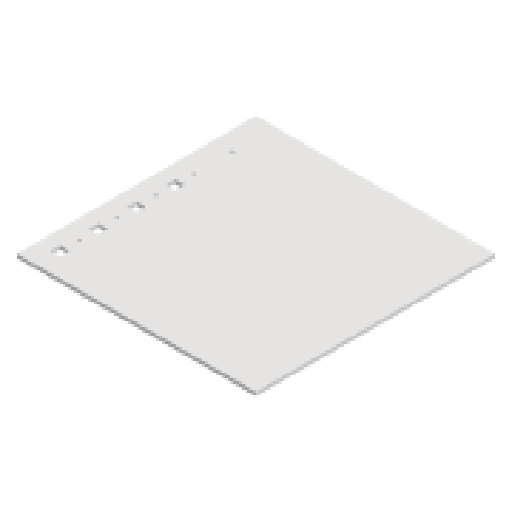
# Autodesk Inventor part: Платформа подъёмника
Saved by Autodesk Inventor 2023.2 (Build 272271030, 271C)
## iProperties
Created: 2025-03-18
Part Number: Платформа подъёмника
Material: Типовые
Document SubType Name: Modeling
Designer: Коноваленко
Density: 1 g/cm^3
Appearance: По умолчанию
Author: Коноваленко
Autodesk Inventor part; units mm, degrees
ref_plane "YZ Plane" through (0, 0, 0) normal (1, 0, 0) x (0, 1, 0)
ref_plane "XZ Plane" through (0, 0, 0) normal (0, 1, 0) x (-1, 0, 0)
ref_plane "XY Plane" through (0, 0, 0) normal (0, 0, 1) x (1, 0, 0)
sketch "Эскиз1" plane through (0, 0, 0) normal (0, 1, 0) x (-1, 0, 0)
  line L0 (125, 125) -> (-125, 125)
  line L1 (-125, 125) -> (-125, -125)
  line L2 (-125, -125) -> (125, -125)
  line L3 (125, -125) -> (125, 125)
  line L4 (125, 125) -> (-125, -125) construction
  line L5 (-125, 125) -> (125, -125) construction
  point P0 (0, 0)
  dimension "d0" = 250
  dimension "d1" = 250
  constraints: 12 end point, 2 midpoint, 2 parallel, 1 horizontal, 1 perpendicular
  measures "d0" distance of L1.end L2.end
  measures "d1" distance of L0.end L1.end
extrude "Выдавливание1" add sketch "Эскиз1" along normal blind 4
sketch "Эскиз2" plane through (0, 0, 0) normal (0, -1, 0) x (1, 0, 0)
  line L0 (-110, 90) -> (-110, 100) projected
  line L1 (-100, 90) -> (-110, 90) projected
  line L2 (-100, 100) -> (-100, 90) projected
  line L3 (-110, 100) -> (-100, 100) projected
  circle A0 centre (-105, 75) radius 2 projected
  circle A1 centre (-105, 35) radius 2 projected
  circle A2 centre (-105, -5) radius 2 projected
  circle A3 centre (-105, -45) radius 2 projected
  circle A4 centre (-105, -85) radius 2 projected
  line L4 (-110, 50) -> (-110, 60) projected
  line L5 (-100, 50) -> (-110, 50) projected
  line L6 (-100, 60) -> (-100, 50) projected
  line L7 (-110, 60) -> (-100, 60) projected
  line L8 (-110, 10) -> (-110, 20) projected
  line L9 (-100, 10) -> (-110, 10) projected
  line L10 (-100, 20) -> (-100, 10) projected
  line L11 (-110, 20) -> (-100, 20) projected
  line L12 (-110, -30) -> (-110, -20) projected
  line L13 (-100, -30) -> (-110, -30) projected
  line L14 (-100, -20) -> (-100, -30) projected
  line L15 (-110, -20) -> (-100, -20) projected
  line L16 (125, 125) -> (125, -125) projected
  line L17 (-125, 125) -> (125, 125) projected
  line L18 (-125, -125) -> (-125, 125) projected
  line L19 (125, -125) -> (-125, -125) projected
  line L20 (110, 90) -> (110, 100) projected
  line L21 (110, 100) -> (100, 100) projected
  line L22 (100, 100) -> (100, 90) projected
  line L23 (100, 90) -> (110, 90) projected
  line L24 (110, 10) -> (110, 20) projected
  line L25 (110, 20) -> (100, 20) projected
  line L26 (100, 20) -> (100, 10) projected
  line L27 (100, 10) -> (110, 10) projected
  line L28 (110, 50) -> (110, 60) projected
  line L29 (110, 60) -> (100, 60) projected
  line L30 (100, 60) -> (100, 50) projected
  line L31 (100, 50) -> (110, 50) projected
  line L32 (110, -30) -> (110, -20) projected
  line L33 (110, -20) -> (100, -20) projected
  line L34 (100, -20) -> (100, -30) projected
  line L35 (100, -30) -> (110, -30) projected
  line L36 (110, -70) -> (110, -60) projected
  line L37 (110, -60) -> (100, -60) projected
  line L38 (100, -60) -> (100, -70) projected
  line L39 (100, -70) -> (110, -70) projected
  line L40 (110, -110) -> (110, -100) projected
  line L41 (110, -100) -> (100, -100) projected
  line L42 (100, -100) -> (100, -110) projected
  line L43 (100, -110) -> (110, -110) projected
  line L44 (-100, -100) -> (-100, -110) projected
  line L45 (-110, -100) -> (-100, -100) projected
  line L46 (-110, -110) -> (-110, -100) projected
  line L47 (-100, -110) -> (-110, -110) projected
  line L48 (-100, -60) -> (-100, -70) projected
  line L49 (-100, -70) -> (-110, -70) projected
  line L50 (-110, -70) -> (-110, -60) projected
  line L51 (-110, -60) -> (-100, -60) projected
  circle A5 centre (105, 75) radius 2 projected
  circle A6 centre (105, 35) radius 2 projected
  circle A7 centre (105, -5) radius 2 projected
  circle A8 centre (105, -45) radius 2 projected
  circle A9 centre (105, -85) radius 2 projected
  point P0 (0, 0)
extrude "Выдавливание2" cut sketch "Эскиз2" against normal up to surface (4 mm away) contours L0 L3 L2 L1 | A0 | A1 | A2 | A3 | A4 | L4 L7 L6 L5 | L8 L11 L10 L9 | L12 L15 L14 L13 | L23 L22 L21 L20 | L27 L26 L25 L24 | L31 L30 L29 L28 | L35 L34 L33 L32 | L39 L38 L37 L36 | L43 L42 L41 L40 | L44 L47 L46 L45 | L48 L49 L50 L51 | A5 | A6 | A7 | A8 | A9
